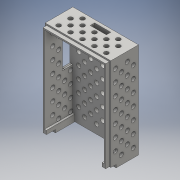
# Autodesk Inventor part: RaspPiCaseBottom
Saved by Autodesk Inventor 2016 (Build 200138000, 138)
## iProperties
Created: 2016-04-29
Part Number: RaspPiCaseBottom
Material: Generic
Document SubType Name: Modeling
Designer: mkepler
Density: 1 g/cm^3
Appearance: Default
Author: mkepler
Autodesk Inventor part; units mm, degrees
ref_plane "YZ Plane" through (0, 0, 0) normal (1, 0, 0) x (0, 1, 0)
ref_plane "XZ Plane" through (0, 0, 0) normal (0, 1, 0) x (-1, 0, 0)
ref_plane "XY Plane" through (0, 0, 0) normal (0, 0, 1) x (1, 0, 0)
sketch "Sketch1" plane through (0, 0, 0) normal (0, 1, 0) x (-1, 0, 0)
  line L0 (0, 0) -> (60, 0)
  line L1 (60, 0) -> (60, -90)
  line L2 (60, -90) -> (0, -90)
  line L3 (0, -90) -> (0, 0)
  circle A0 centre (6, -6) radius 2.15
  circle A1 centre (12, -12) radius 2.15
  line L4 (0, 0) -> (15, 0)
  line L5 (15, -28.7108) -> (16.2859, -28.7108)
  circle A2 centre (24, -12) radius 2.15
  circle A3 centre (18, -6) radius 2.15
  line L6 (0, 0) -> (27, 0)
  circle A4 centre (48, -12) radius 2.15
  circle A5 centre (42, -6) radius 2.15
  circle A6 centre (30, -6) radius 2.15
  circle A7 centre (36, -12) radius 2.15
  circle A8 centre (54, -6) radius 2.15
  line L7 (60, 0) -> (60, -15)
  line L8 (60, 0) -> (60, -15)
  line L9 (60, -15) -> (56.15, -15)
  circle A9 centre (6, -18) radius 2.15
  circle A10 centre (12, -24) radius 2.15
  circle A11 centre (24, -24) radius 2.15
  circle A12 centre (18, -18) radius 2.15
  circle A13 centre (30, -18) radius 2.15
  circle A14 centre (36, -24) radius 2.15
  circle A15 centre (42, -18) radius 2.15
  circle A16 centre (48, -24) radius 2.15
  circle A17 centre (54, -18) radius 2.15
  line L10 (60, 0) -> (60, -27)
  circle A18 centre (6, -42) radius 2.15
  circle A19 centre (18, -42) radius 2.15
  circle A20 centre (30, -42) radius 2.15
  circle A21 centre (42, -42) radius 2.15
  circle A22 centre (54, -42) radius 2.15
  circle A23 centre (54, -30) radius 2.15
  circle A24 centre (48, -36) radius 2.15
  circle A25 centre (42, -30) radius 2.15
  circle A26 centre (36, -36) radius 2.15
  circle A27 centre (30, -30) radius 2.15
  circle A28 centre (24, -36) radius 2.15
  circle A29 centre (18, -30) radius 2.15
  circle A30 centre (12, -36) radius 2.15
  circle A31 centre (6, -30) radius 2.15
  line L11 (60, 0) -> (60, -45)
  line L12 (60, -45) -> (48.8128, -45)
  circle A32 centre (6, -78) radius 2.15
  circle A33 centre (12, -84) radius 2.15
  line L13 (15, -61.2892) -> (16.2859, -61.2892)
  circle A34 centre (24, -84) radius 2.15
  circle A35 centre (18, -78) radius 2.15
  circle A36 centre (30, -78) radius 2.15
  circle A37 centre (36, -84) radius 2.15
  circle A38 centre (42, -78) radius 2.15
  circle A39 centre (48, -84) radius 2.15
  circle A40 centre (54, -78) radius 2.15
  line L14 (60, -75) -> (56.15, -75)
  circle A41 centre (54, -66) radius 2.15
  circle A42 centre (48, -72) radius 2.15
  circle A43 centre (42, -66) radius 2.15
  circle A44 centre (36, -72) radius 2.15
  circle A45 centre (30, -66) radius 2.15
  circle A46 centre (24, -72) radius 2.15
  circle A47 centre (18, -66) radius 2.15
  circle A48 centre (12, -72) radius 2.15
  circle A49 centre (6, -66) radius 2.15
  circle A50 centre (54, -54) radius 2.15
  circle A51 centre (48, -60) radius 2.15
  circle A52 centre (48, -48) radius 2.15
  circle A53 centre (42, -54) radius 2.15
  circle A54 centre (36, -60) radius 2.15
  circle A55 centre (36, -48) radius 2.15
  circle A56 centre (30, -54) radius 2.15
  circle A57 centre (24, -60) radius 2.15
  circle A58 centre (24, -48) radius 2.15
  circle A59 centre (18, -54) radius 2.15
  circle A60 centre (12, -60) radius 2.15
  circle A61 centre (12, -48) radius 2.15
  circle A62 centre (6, -54) radius 2.15
  dimension "d0" = 60
  dimension "d1" = 4.3
  dimension "d2" = 6
  dimension "d3" = 6
  dimension "d6" = 90
  dimension "d7" = 4.3
  dimension "d10" = 15
  dimension "d12" = 27
  dimension "d13" = 4.3
  dimension "d17" = 15
  dimension "d18" = 27
  dimension "d19" = 45
  constraints: 63 centre point, 30 end point, 4 point on line, 4 symmetric about line, 2 horizontal, 2 parallel, 2 perpendicular, 1 collinear, 1 midpoint
  measures "d0" distance of L1.end L2.end
  measures "d1" diameter of A0
  measures "d2" distance from line of L0 A0.centre
  measures "d3" distance from line of L3 A0.centre
  measures "d6" distance of L0.end L1.end
  measures "d7" diameter of A1
  measures "d10" distance of L0.start L4.end
  measures "d12" distance of L0.start L6.end
  measures "d13" diameter of A8
  measures "d17" distance of L0.end L7.end
  measures "d18" distance of L0.end L10.end
  measures "d19" distance of L0.end L11.end
extrude "Extrusion1" add sketch "Sketch1" along normal blind 1.5
sketch "Sketch3" plane through (0, 0, 0) normal (1, 0, 0) x (0, 0, -1)
  line L0 (0, 1.5) -> (90, 1.5) projected
  line L1 (0, 1.5) -> (90, 1.5)
  line L2 (90, 1.5) -> (90, -28.5)
  line L3 (90, -28.5) -> (0, -28.5)
  line L4 (0, -28.5) -> (0, 1.5)
  point P0 (0, 0)
  dimension "d25" = 90
  dimension "d26" = 30
  constraints: 8 end point, 2 parallel, 1 horizontal, 1 perpendicular
  measures "d25" distance of L2.end L3.end
  measures "d26" distance of L1.end L2.end
extrude "Extrusion3" add sketch "Sketch3" along normal blind 1.5
sketch "Sketch5" plane through (-60, 0, -90) normal (-1, 0, 0) x (0, 0, 1)
  line L0 (90, -28.5) -> (90, 0) projected
  line L1 (90, 1.5) -> (0, 1.5)
  line L2 (0, 1.5) -> (0, -28.5)
  line L3 (0, -28.5) -> (90, -28.5)
  line L4 (90, -28.5) -> (90, 1.5)
  dimension "d31" = 90
  dimension "d32" = 30
  constraints: 8 end point, 2 parallel, 1 horizontal, 1 perpendicular
  measures "d31" distance of L3.end L2.end
  measures "d32" distance of L2.end L1.end
extrude "Extrusion5" add sketch "Sketch5" along normal blind 1.5
sketch "Sketch8" plane through (0, 1.5, 0) normal (0, 1, 0) x (1, 0, 0)
  line L0 (-61.5, 0) -> (-61.5, 90) projected
  line L1 (-61.5, 0) -> (1.5, 0)
  line L2 (1.5, 0) -> (1.5, -1.5)
  line L3 (1.5, -1.5) -> (-61.5, -1.5)
  line L4 (-61.5, -1.5) -> (-61.5, 0)
  point P0 (0, 0)
  dimension "d40" = 63
  dimension "d41" = 1.5
  constraints: 8 end point, 2 parallel, 1 horizontal, 1 perpendicular
  measures "d40" distance of L2.end L3.end
  measures "d41" distance of L1.end L2.end
extrude "Extrusion7" add sketch "Sketch8" against normal blind 30
sketch "Sketch9" plane through (-61.5, 0, -90) normal (-1, 0, 0) x (0, 0, 1)
  line L0 (91.5, 1.5) -> (91.5, -28.5) projected
  circle A0 centre (84, -8.3) radius 2.15
  line L1 (84, -2.3) -> (84, -8.3)
  line L2 (91.5, 1.5) -> (91.5, -28.5) projected
  line L3 (84, -8.3) -> (84, -11.3)
  line L4 (84, -11.3) -> (91.5, -11.3)
  circle A1 centre (84, -20.3) radius 2.15
  line L5 (84, -20.3) -> (84, -14.3)
  line L6 (84, -14.3) -> (84, -11.3)
  line L7 (81, -2.3) -> (81, -28.5)
  circle A2 centre (78, -2.3) radius 2.15
  line L8 (78, -2.3) -> (78, -8.3)
  line L9 (78, -8.3) -> (78, -11.3)
  line L10 (78, -11.3) -> (70.5, -11.3)
  circle A3 centre (78, -14.3) radius 2.15
  line L11 (78, -20.3) -> (78, -14.3)
  line L12 (78, -14.3) -> (78, -11.3)
  line L13 (78, -2.3) -> (81, -2.3)
  line L14 (78, -20.3) -> (75, -20.3)
  line L15 (75, -20.3) -> (75, -8.9833)
  circle A4 centre (66, -2.3) radius 2.15
  line L16 (66, -11.3) -> (58.5, -11.3)
  circle A5 centre (66, -14.3) radius 2.15
  line L17 (69, -2.3) -> (69, -28.5)
  line L18 (72, -11.3) -> (79.5, -11.3)
  circle A6 centre (72, -8.3) radius 2.15
  circle A7 centre (72, -20.3) radius 2.15
  line L19 (72, -20.3) -> (75, -20.3)
  line L20 (66, -20.3) -> (63, -20.3)
  line L21 (63, -20.3) -> (63, -15.4)
  circle A8 centre (42, -2.3) radius 2.15
  line L22 (42, -2.3) -> (42, -8.3)
  line L23 (42, -8.3) -> (42, -11.3)
  circle A9 centre (42, -14.3) radius 2.15
  line L24 (42, -20.3) -> (42, -14.3)
  line L25 (42, -14.3) -> (42, -11.3)
  line L26 (42, -2.3) -> (45, -2.3)
  line L27 (48, -2.3) -> (48, -8.3)
  line L28 (48, -2.3) -> (45, -2.3)
  line L29 (48, -11.3) -> (55.5, -11.3)
  line L30 (48, -8.3) -> (48, -11.3)
  circle A10 centre (48, -8.3) radius 2.15
  line L31 (48, -14.3) -> (48, -11.3)
  line L32 (48, -20.3) -> (48, -14.3)
  circle A11 centre (48, -20.3) radius 2.15
  line L33 (48, -20.3) -> (51, -20.3)
  line L34 (51, -20.3) -> (51, -8.9833)
  circle A12 centre (54, -14.3) radius 2.15
  line L35 (54, -20.3) -> (51, -20.3)
  circle A13 centre (60, -20.3) radius 2.15
  circle A14 centre (60, -8.3) radius 2.15
  line L36 (54, -11.3) -> (46.5, -11.3)
  circle A15 centre (54, -2.3) radius 2.15
  line L37 (42, -20.3) -> (39, -20.3)
  line L38 (39, -20.3) -> (39, -14.6416)
  circle A16 centre (6, -14.3) radius 2.15
  circle A17 centre (12, -20.3) radius 2.15
  circle A18 centre (12, -8.3) radius 2.15
  circle A19 centre (6, -2.3) radius 2.15
  line L39 (12, -20.3) -> (15, -20.3)
  line L40 (15, -20.3) -> (15, -15.4)
  circle A20 centre (24, -20.3) radius 2.15
  line L41 (30, -20.3) -> (27, -20.3)
  line L42 (30, -20.3) -> (30, -14.3)
  line L43 (30, -11.3) -> (22.5, -11.3)
  line L44 (30, -14.3) -> (30, -11.3)
  line L45 (24, -11.3) -> (31.5, -11.3)
  circle A21 centre (30, -14.3) radius 2.15
  line L46 (30, -8.3) -> (30, -11.3)
  line L47 (36, -20.3) -> (36, -14.3)
  circle A22 centre (36, -20.3) radius 2.15
  line L48 (24, -20.3) -> (27, -20.3)
  line L49 (30, -2.3) -> (30, -8.3)
  line L50 (30, -2.3) -> (33, -2.3)
  circle A23 centre (30, -2.3) radius 2.15
  circle A24 centre (36, -8.3) radius 2.15
  line L51 (36, -2.3) -> (36, -8.3)
  line L52 (36, -8.3) -> (36, -11.3)
  line L53 (36, -14.3) -> (36, -11.3)
  line L54 (36, -2.3) -> (33, -2.3)
  circle A25 centre (24, -8.3) radius 2.15
  circle A26 centre (18, -2.3) radius 2.15
  circle A27 centre (18, -14.3) radius 2.15
  line L55 (36, -20.3) -> (39, -20.3)
  point P0 (90, 0)
  point P1 (66, -8.3)
  point P2 (72, -2.3)
  point P3 (60, -2.3)
  point P4 (60, -14.3)
  point P5 (57, -2.3)
  point P6 (60, -11.3)
  point P7 (54, -8.3)
  point P8 (12, -2.3)
  point P9 (12, -14.3)
  point P10 (6, -20.3)
  point P11 (6, -8.3)
  point P12 (18, -20.3)
  point P13 (24, -14.3)
  point P14 (18, -11.3)
  point P15 (18, -8.3)
  point P16 (24, -2.3)
  point P17 (21, -2.3)
  dimension "d46" = 7.5
  dimension "d47" = 4.3
  dimension "d48" = 6
  dimension "d49" = 3
  dimension "d50" = 3
  dimension "d51" = 3
  dimension "d52" = 3
  dimension "d53" = 3
  constraints: 108 end point, 80 symmetric about line, 28 centre point, 13 point on line, 3 horizontal, 3 perpendicular, 1 parallel, 1 vertical
  measures "d46" distance from line of L0 L1.start
  measures "d47" diameter of A0
  measures "d48" distance of L1.start L1.end
  measures "d49" distance of L1.end L3.end
  measures "d50" distance of L1.start L7.start
  measures "d51" distance of L11.start L14.end
  measures "d52" distance of L20.start L20.end
  measures "d53" distance of L24.start L37.end
sketch "Sketch10" plane through (-61.5, 1.5, 1.5) normal (0, 0, 1) x (1, 0, 0)
  line L0 (63, 0) -> (0, 0) projected
  line L1 (0, 0) -> (0, -30) projected
  circle A0 centre (13.5, -3.8) radius 2.15
  circle A1 centre (7.5, -9.8) radius 2.15
  line L2 (7.5, -9.8) -> (7.5, -12.8)
  line L3 (7.5, -12.8) -> (8.9551, -12.8)
  circle A2 centre (7.5, -21.8) radius 2.15
  circle A3 centre (13.5, -15.8) radius 2.15
  line L4 (7.5, -15.8) -> (7.5, -12.8)
  line L5 (13.5, -3.8) -> (16.5, -3.8)
  line L6 (16.5, -3.8) -> (16.5, -8.3155)
  circle A4 centre (25.5, -3.8) radius 2.15
  circle A5 centre (19.5, -9.8) radius 2.15
  line L7 (25.5, -9.8) -> (25.5, -12.8)
  line L8 (25.5, -12.8) -> (24.0449, -12.8)
  circle A6 centre (19.5, -21.8) radius 2.15
  circle A7 centre (25.5, -15.8) radius 2.15
  line L9 (25.5, -15.8) -> (25.5, -12.8)
  line L10 (19.5, -3.8) -> (16.5, -3.8)
  line L11 (25.5, -3.8) -> (28.5, -3.8)
  line L12 (28.5, -3.8) -> (28.5, -7.65)
  circle A8 centre (49.5, -3.8) radius 2.15
  circle A9 centre (43.5, -9.8) radius 2.15
  line L13 (49.5, -9.8) -> (49.5, -12.8)
  line L14 (49.5, -12.8) -> (48.0449, -12.8)
  circle A10 centre (43.5, -21.8) radius 2.15
  circle A11 centre (49.5, -15.8) radius 2.15
  line L15 (49.5, -15.8) -> (49.5, -12.8)
  line L16 (43.5, -3.8) -> (40.5, -3.8)
  line L17 (40.5, -3.8) -> (40.5, -8.3155)
  line L18 (31.5, -12.8) -> (32.9551, -12.8)
  line L19 (31.5, -15.8) -> (31.5, -12.8)
  circle A12 centre (37.5, -15.8) radius 2.15
  circle A13 centre (31.5, -21.8) radius 2.15
  line L20 (31.5, -9.8) -> (31.5, -12.8)
  circle A14 centre (31.5, -9.8) radius 2.15
  line L21 (37.5, -3.8) -> (40.5, -3.8)
  circle A15 centre (37.5, -3.8) radius 2.15
  line L22 (49.5, -3.8) -> (52.5, -3.8)
  line L23 (52.5, -3.8) -> (52.5, -9.251)
  circle A16 centre (55.5, -9.8) radius 2.15
  line L24 (55.5, -9.8) -> (55.5, -12.8)
  line L25 (55.5, -12.8) -> (56.9551, -12.8)
  circle A17 centre (55.5, -21.8) radius 2.15
  line L26 (55.5, -15.8) -> (55.5, -12.8)
  line L27 (55.5, -3.8) -> (52.5, -3.8)
  point P0 (61.5, -1.5)
  point P1 (7.5, -3.8)
  point P2 (13.5, -9.8)
  point P3 (13.5, -21.8)
  point P4 (25.5, -21.8)
  point P5 (19.5, -15.8)
  point P6 (43.5, -15.8)
  point P7 (37.5, -21.8)
  point P8 (37.5, -9.8)
  point P9 (31.5, -3.8)
  dimension "d62" = 3.8
  dimension "d63" = 7.5
  dimension "d64" = 4.3
  dimension "d65" = 6
  dimension "d66" = 4.3
  dimension "d67" = 6
  dimension "d69" = 3
  dimension "d70" = 3
  dimension "d71" = 3
  dimension "d72" = 3
  constraints: 52 end point, 40 symmetric about line, 18 centre point, 4 horizontal, 3 perpendicular, 1 vertical
  measures "d62" distance from line of L0 point (7.5, -3.8)
  measures "d63" distance from line of L1 point (7.5, -3.8)
  measures "d64" diameter of A0
  measures "d65" distance of L5.start point (7.5, -3.8)
  measures "d66" diameter of A1
  measures "d67" distance of L2.start point (7.5, -3.8)
  measures "d69" distance of L2.start L2.end
  measures "d70" distance of L5.start L5.end
  measures "d71" distance of L11.start L11.end
  measures "d72" distance of L22.start L22.end
sketch "Sketch11" plane through (-61.5, 1.5, 1.5) normal (0, 0, 1) x (1, 0, 0)
  line L0 (1.5, -1.5) -> (61.5, -1.5) projected
  line L1 (39.65, -1.5) -> (23.1579, -1.5)
  line L2 (23.1579, -1.5) -> (23.1579, -5.95)
  line L3 (23.1579, -5.95) -> (39.65, -5.95)
  line L4 (39.65, -5.95) -> (39.65, -1.5)
  constraints: 8 end point, 2 parallel, 1 horizontal, 1 perpendicular, 1 point on line
extrude "Extrusion8" cut sketch "Sketch11" against normal blind 30
sketch "Sketch12" plane through (-60, 0, -90) normal (1, 0, 0) x (0, 0, -1)
  line L0 (0, 0) -> (-90, 0) projected
  line L1 (0, -28.5) -> (-90, -28.5) projected
  line L2 (0, 0) -> (-3.7, 0)
  line L3 (-3.7, 0) -> (-3.7, -28.5)
  line L4 (-3.7, -28.5) -> (0, -28.5)
  line L5 (0, -28.5) -> (0, 0)
  dimension "d82" = 3.7
  constraints: 8 end point, 2 parallel, 1 horizontal, 1 perpendicular, 1 point on line
  measures "d82" distance of L4.end L3.end
extrude "Extrusion9" add sketch "Sketch12" along normal blind 2
sketch "Sketch13" plane through (0, 0, 0) normal (-1, 0, 0) x (0, 0, 1)
  line L0 (-90, -28.5) -> (0, -28.5) projected
  line L1 (-90, 0) -> (-86.3, 0)
  line L2 (-86.3, 0) -> (-86.3, -28.5)
  line L3 (-86.3, -28.5) -> (-90, -28.5)
  line L4 (-90, -28.5) -> (-90, 0)
  point P0 (0, 0)
  dimension "d85" = 3.7
  constraints: 8 end point, 2 parallel, 1 horizontal, 1 perpendicular, 1 point on line
  measures "d85" distance of L2.end L3.end
extrude "Extrusion10" add sketch "Sketch13" along normal blind 2
sketch "Sketch14" plane through (0, 0, 0) normal (-1, 0, 0) x (0, 0, 1)
  point P0 (0, 0)
sketch "Sketch16" plane through (0, 0, 0) normal (0, -1, 0) x (1, 0, 0)
  point P0 (0, 0)
hole "Hole3" at (-61.5, -20.3, -6) at (-61.5, -14.3, -12) at (-61.5, -20.3, -18) at (-61.5, -14.3, -24) at (-61.5, -8.3, -6) at (-61.5, -2.3, -12) at (-61.5, -8.3, -18) at (-61.5, -2.3, -24) at (-61.5, -8.3, -30) at (-61.5, -20.3, -30) at (-61.5, -14.3, -36) at (-61.5, -2.3, -36) at (-61.5, -8.3, -42) at (-61.5, -20.3, -42) at (-61.5, -14.3, -48) at (-61.5, -20.3, -54) at (-61.5, -8.3, -54) at (-61.5, -2.3, -48) at (-61.5, -2.3, -60) at (-61.5, -14.3, -60) at (-61.5, -8.3, -66) at (-61.5, -8.3, -78) at (-61.5, -14.3, -72) at (-61.5, -20.3, -66) at (-61.5, -2.3, -72) at (-61.5, -2.3, -84) at (-61.5, -14.3, -84) at (-61.5, -20.3, -78) direction (1, 0, 0) diameter 4.35 end through all
hole "Hole4" at (-6, -20.3, 1.5) at (-18, -20.3, 1.5) at (-30, -20.3, 1.5) at (-42, -20.3, 1.5) at (-54, -20.3, 1.5) at (-48, -14.3, 1.5) at (-36, -14.3, 1.5) at (-24, -14.3, 1.5) at (-12, -14.3, 1.5) at (-6, -8.3, 1.5) at (-18, -8.3, 1.5) at (-12, -2.3, 1.5) at (-30, -8.3, 1.5) at (-42, -8.3, 1.5) at (-48, -2.3, 1.5) at (-54, -8.3, 1.5) direction (0, 0, -1) diameter 4.35 end through all
sketch "Sketch17" plane through (-61.5, 0, -90) normal (-1, 0, 0) x (0, 0, 1)
  line L0 (86.15, 0) -> (81.85, 0) projected
  line L1 (86.15, 0) -> (86.15, -10.475)
  line L2 (86.15, -10.475) -> (45.825, -10.475)
  line L3 (45.825, -10.475) -> (45.85, 0)
  line L4 (45.85, 0) -> (45.85, 1.5) projected
  line L5 (50.15, 0) -> (45.85, 0) projected
  line L6 (86.15, 0) -> (45.85, 0)
  point P0 (90, 0)
  constraints: 8 end point, 1 horizontal, 1 perpendicular, 1 point on line, 1 vertical
extrude "Extrusion12" cut sketch "Sketch17" against normal blind 10
sketch "Sketch18" plane through (-61.5, 0, -90) normal (-1, 0, 0) x (0, 0, 1)
  line L0 (91.5, 1.5) -> (91.5, -28.5) projected
  line L1 (91.5, -28.5) -> (91.5, -24.85)
  line L2 (91.5, -24.85) -> (0, -24.85)
  line L3 (0, -28.5) -> (0, 0) projected
  line L4 (91.5, 1.5) -> (0, 1.5) projected
  line L5 (0, 1.5) -> (91.5, 1.5)
  line L6 (91.5, 1.5) -> (91.5, -24.85)
  line L7 (0, 1.5) -> (0, -24.85)
  circle A0 centre (84, -20.3) radius 2.175 projected
  circle A1 centre (84, -20.3) radius 2.175
  circle A2 centre (66, -14.3) radius 2.175 projected
  circle A3 centre (66, -14.3) radius 2.175
  circle A4 centre (72, -20.3) radius 2.175 projected
  circle A5 centre (72, -20.3) radius 2.175
  circle A6 centre (60, -20.3) radius 2.175 projected
  circle A7 centre (60, -20.3) radius 2.175
  circle A8 centre (54, -14.3) radius 2.175 projected
  circle A9 centre (54, -14.3) radius 2.175
  circle A10 centre (48, -20.3) radius 2.175 projected
  circle A11 centre (48, -20.3) radius 2.175
  circle A12 centre (36, -20.3) radius 2.175 projected
  circle A13 centre (36, -20.3) radius 2.175
  circle A14 centre (42, -14.3) radius 2.175 projected
  circle A15 centre (42, -14.3) radius 2.175
  circle A16 centre (78, -14.3) radius 2.175 projected
  circle A17 centre (78, -14.3) radius 2.175
  circle A18 centre (42, -2.3) radius 2.175 projected
  circle A19 centre (42, -2.3) radius 2.175
  circle A20 centre (36, -8.3) radius 2.175 projected
  circle A21 centre (36, -8.3) radius 2.175
  circle A22 centre (30, -2.3) radius 2.175 projected
  circle A23 centre (30, -2.3) radius 2.175
  circle A24 centre (24, -8.3) radius 2.175 projected
  circle A25 centre (24, -8.3) radius 2.175
  circle A26 centre (24, -20.3) radius 2.175 projected
  circle A27 centre (24, -20.3) radius 2.175
  circle A28 centre (6, -14.3) radius 2.175 projected
  circle A29 centre (6, -14.3) radius 2.175
  circle A30 centre (12, -8.3) radius 2.175 projected
  circle A31 centre (12, -8.3) radius 2.175
  circle A32 centre (6, -2.3) radius 2.175
  circle A33 centre (18, -2.3) radius 2.175
  line L8 (90, 0) -> (3.7, 0) projected
  line L9 (86.175, 0) -> (45.825, 0)
  line L10 (45.825, 0) -> (45.825, -10.475)
  line L11 (45.825, -10.475) -> (86.175, -10.475)
  line L12 (86.175, -10.475) -> (86.175, 0)
  circle A34 centre (30, -14.3) radius 2.175
  circle A35 centre (18, -14.3) radius 2.175
  circle A36 centre (12, -20.3) radius 2.175
  dimension "d116" = 3.65
  dimension "d117" = 4.35
  dimension "d118" = 4.35
  dimension "d119" = 4.35
  dimension "d120" = 4.35
  dimension "d121" = 4.35
  dimension "d122" = 4.35
  dimension "d123" = 4.35
  dimension "d124" = 4.35
  dimension "d125" = 4.35
  dimension "d126" = 4.35
  constraints: 21 centre point, 18 end point, 16 coincident, 3 perpendicular, 3 point on line, 2 collinear, 2 parallel, 1 horizontal
  measures "d116" distance of L0.end L1.end
  measures "d117" diameter of A1
  measures "d118" diameter of A3
  measures "d119" diameter of A5
  measures "d120" diameter of A7
  measures "d121" diameter of A9
  measures "d122" diameter of A11
  measures "d123" diameter of A13
  measures "d124" diameter of A15
  measures "d125" diameter of A23
  measures "d126" diameter of A25
extrude "Extrusion13" add sketch "Sketch18" along normal blind 1.5
sketch "Sketch19" plane through (-61.5, -28.5, 1.5) normal (0, 0, 1) x (1, 0, 0)
  point P0 (61.5, 28.5)
sketch "Sketch20" plane through (1.5, 0, 0) normal (1, 0, 0) x (0, 0, -1)
  line L0 (-1.5, -24.85) -> (90, -24.85) projected
  line L1 (-1.5, -24.85) -> (-1.5, -28.5) projected
  line L2 (90, -24.85) -> (-1.5, -24.85)
  line L3 (-1.5, -24.85) -> (-1.5, 1.5) projected
  line L4 (-1.5, -24.85) -> (-1.5, 1.5)
  line L5 (-1.5, 1.5) -> (90, 1.5) projected
  line L6 (-1.5, 1.5) -> (90, 1.5)
  line L7 (90, 1.5) -> (90, -24.85)
  line L8 (90, -28.5) -> (90, 0) projected
  circle A0 centre (78.0652, -20.3438) radius 2.175
  circle A1 centre (84, -14.3) radius 2.175 projected
  circle A2 centre (84, -14.3) radius 2.175
  circle A3 centre (72, -2.3) radius 2.175 projected
  circle A4 centre (72, -2.3) radius 2.175
  circle A5 centre (84, -2.3) radius 2.175
  circle A6 centre (72, -14.3) radius 2.175
  circle A7 centre (66, -20.3) radius 2.175 projected
  circle A8 centre (66, -20.3) radius 2.175
  circle A9 centre (66, -8.3) radius 2.175
  circle A10 centre (60, -2.3) radius 2.175 projected
  circle A11 centre (60, -2.3) radius 2.175
  circle A12 centre (60, -14.3) radius 2.175 projected
  circle A13 centre (60, -14.3) radius 2.175
  circle A14 centre (54, -20.3) radius 2.175 projected
  circle A15 centre (54, -20.3) radius 2.175
  circle A16 centre (54, -8.3) radius 2.175
  circle A17 centre (48, -2.3) radius 2.175 projected
  circle A18 centre (48, -2.3) radius 2.175
  circle A19 centre (48, -14.3) radius 2.175
  circle A20 centre (42, -20.3) radius 2.175 projected
  circle A21 centre (42, -20.3) radius 2.175
  circle A22 centre (42, -8.3) radius 2.175 projected
  circle A23 centre (42, -8.3) radius 2.175
  circle A24 centre (36, -2.3) radius 2.175 projected
  circle A25 centre (36, -2.3) radius 2.175
  circle A26 centre (30, -20.3) radius 2.175 projected
  circle A27 centre (30, -20.3) radius 2.175
  circle A28 centre (36, -14.3) radius 2.175 projected
  circle A29 centre (36, -14.3) radius 2.175
  circle A30 centre (30, -8.3) radius 2.175
  circle A31 centre (24, -14.3) radius 2.175 projected
  circle A32 centre (24, -14.3) radius 2.175
  circle A33 centre (24, -2.3) radius 2.175
  circle A34 centre (6, -8.3) radius 2.175 projected
  circle A35 centre (6, -8.3) radius 2.175
  circle A36 centre (12, -2.3) radius 2.175 projected
  circle A37 centre (12, -2.3) radius 2.175
  circle A38 centre (18, -8.3) radius 2.175 projected
  circle A39 centre (18, -8.3) radius 2.175
  circle A40 centre (12, -14.3) radius 2.175
  circle A41 centre (6, -20.3) radius 2.175
  circle A42 centre (18, -20.3) radius 2.175
  point P0 (0, 0)
  dimension "d129" = 4.35
  dimension "d130" = 4.35
  constraints: 27 centre point, 16 coincident, 8 end point, 3 collinear, 1 perpendicular
  measures "d129" diameter of A0
  measures "d130" diameter of A2
extrude "Extrusion14" add sketch "Sketch20" along normal blind 1.5
sketch "Sketch21" plane through (-61.5, -28.5, 1.5) normal (0, 0, 1) x (1, 0, 0)
  line L0 (63, 3.65) -> (64.5, 3.65) projected
  line L1 (0, 3.65) -> (-1.5, 3.65) projected
  line L2 (64.5, 3.65) -> (-1.5, 3.65)
  line L3 (-1.5, 3.65) -> (-1.5, 30) projected
  line L4 (-1.5, 3.65) -> (-1.5, 30)
  line L5 (-1.5, 30) -> (64.5, 30) projected
  line L6 (-1.5, 30) -> (64.5, 30)
  line L7 (64.5, 30) -> (64.5, 3.65) projected
  line L8 (64.5, 30) -> (64.5, 3.65)
  circle A0 centre (55.5, 8.2) radius 2.175 projected
  circle A1 centre (55.5, 8.2) radius 2.175
  circle A2 centre (49.5, 14.2) radius 2.175 projected
  circle A3 centre (49.5, 14.2) radius 2.175
  circle A4 centre (55.5, 20.2) radius 2.175 projected
  circle A5 centre (55.5, 20.2) radius 2.175
  circle A6 centre (49.5, 26.2) radius 2.175 projected
  circle A7 centre (49.5, 26.2) radius 2.175
  circle A8 centre (43.5, 20.2) radius 2.175 projected
  circle A9 centre (43.5, 20.2) radius 2.175
  circle A10 centre (43.5, 8.2) radius 2.175 projected
  circle A11 centre (43.5, 8.2) radius 2.175
  circle A12 centre (37.5, 14.2) radius 2.175 projected
  circle A13 centre (37.5, 14.2) radius 2.175
  circle A14 centre (31.5, 8.2) radius 2.175
  circle A15 centre (31.5, 20.2) radius 2.175
  circle A16 centre (19.5, 20.2) radius 2.175 projected
  circle A17 centre (19.5, 20.2) radius 2.175
  circle A18 centre (25.5, 14.2) radius 2.175 projected
  circle A19 centre (25.5, 14.2) radius 2.175
  circle A20 centre (7.5, 8.2) radius 2.175 projected
  circle A21 centre (7.5, 8.2) radius 2.175
  circle A22 centre (13.5, 14.2) radius 2.175 projected
  circle A23 centre (13.5, 14.2) radius 2.175
  circle A24 centre (7.5, 20.2) radius 2.175
  circle A25 centre (13.5, 26.2) radius 2.175
  line L9 (23.1579, 24.05) -> (39.65, 24.05) projected
  line L10 (27.65, 28.5) -> (23.35, 28.5) projected
  line L11 (39.65, 24.05) -> (23.35, 24.05)
  line L12 (23.35, 24.05) -> (23.35, 28.5)
  line L13 (23.35, 28.5) -> (39.65, 28.5)
  line L14 (39.65, 28.5) -> (39.65, 24.05)
  circle A26 centre (19.5, 8.2) radius 2.175
  point P0 (61.5, 28.5)
  constraints: 16 centre point, 16 end point, 11 coincident, 3 equal length, 3 perpendicular, 2 horizontal
sketch "Sketch22" plane through (0, 1.5, 0) normal (0, 1, 0) x (1, 0, 0)
  line L0 (1.5, 90) -> (3, 90) projected
  line L1 (-63, -3) -> (3, -3)
  line L2 (3, -3) -> (3, 90)
  line L3 (3, 90) -> (-63, 90)
  line L4 (-63, 90) -> (-63, -3)
  circle A0 centre (-54, 6) radius 2.15 projected
  circle A1 centre (-54, 6) radius 2.15
  circle A2 centre (-54, 18) radius 2.15 projected
  circle A3 centre (-54, 18) radius 2.15
  circle A4 centre (-54, 30) radius 2.15 projected
  circle A5 centre (-54, 30) radius 2.15
  circle A6 centre (-54, 54) radius 2.15 projected
  circle A7 centre (-54, 54) radius 2.15
  circle A8 centre (-54, 66) radius 2.15 projected
  circle A9 centre (-54, 66) radius 2.15
  circle A10 centre (-54, 78) radius 2.15 projected
  circle A11 centre (-54, 78) radius 2.15
  circle A12 centre (-48, 84) radius 2.15 projected
  circle A13 centre (-48, 84) radius 2.15
  circle A14 centre (-48, 72) radius 2.15 projected
  circle A15 centre (-48, 72) radius 2.15
  circle A16 centre (-48, 60) radius 2.15 projected
  circle A17 centre (-48, 60) radius 2.15
  circle A18 centre (-48, 48) radius 2.15 projected
  circle A19 centre (-48, 48) radius 2.15
  circle A20 centre (-48, 36) radius 2.15 projected
  circle A21 centre (-48, 36) radius 2.15
  circle A22 centre (-48, 24) radius 2.15 projected
  circle A23 centre (-48, 24) radius 2.15
  circle A24 centre (-48, 12) radius 2.15 projected
  circle A25 centre (-48, 12) radius 2.15
  circle A26 centre (-42, 6) radius 2.15 projected
  circle A27 centre (-42, 6) radius 2.15
  circle A28 centre (-42, 18) radius 2.15 projected
  circle A29 centre (-42, 18) radius 2.15
  circle A30 centre (-42, 30) radius 2.15 projected
  circle A31 centre (-42, 30) radius 2.15
  circle A32 centre (-54, 42) radius 2.15 projected
  circle A33 centre (-54, 42) radius 2.15
  circle A34 centre (-42, 42) radius 2.15 projected
  circle A35 centre (-42, 42) radius 2.15
  circle A36 centre (-42, 54) radius 2.15
  circle A37 centre (-42, 66) radius 2.15 projected
  circle A38 centre (-42, 66) radius 2.15
  circle A39 centre (-42, 78) radius 2.15 projected
  circle A40 centre (-42, 78) radius 2.15
  circle A41 centre (-36, 12) radius 2.15 projected
  circle A42 centre (-36, 12) radius 2.15
  circle A43 centre (-24, 12) radius 2.15 projected
  circle A44 centre (-24, 12) radius 2.15
  circle A45 centre (-30, 6) radius 2.15
  circle A46 centre (-30, 18) radius 2.15 projected
  circle A47 centre (-30, 18) radius 2.15
  circle A48 centre (-36, 24) radius 2.15 projected
  circle A49 centre (-36, 24) radius 2.15
  circle A50 centre (-36, 36) radius 2.15 projected
  circle A51 centre (-36, 36) radius 2.15
  circle A52 centre (-36, 48) radius 2.15 projected
  circle A53 centre (-36, 48) radius 2.15
  circle A54 centre (-36, 60) radius 2.15 projected
  circle A55 centre (-36, 60) radius 2.15
  circle A56 centre (-36, 72) radius 2.15
  circle A57 centre (-36, 84) radius 2.15
  circle A58 centre (-30, 78) radius 2.15 projected
  circle A59 centre (-30, 78) radius 2.15
  circle A60 centre (-30, 66) radius 2.15 projected
  circle A61 centre (-30, 66) radius 2.15
  circle A62 centre (-30, 54) radius 2.15 projected
  circle A63 centre (-30, 54) radius 2.15
  circle A64 centre (-30, 42) radius 2.15
  circle A65 centre (-30, 30) radius 2.15 projected
  circle A66 centre (-30, 30) radius 2.15
  circle A67 centre (-24, 24) radius 2.15 projected
  circle A68 centre (-24, 24) radius 2.15
  circle A69 centre (-24, 48) radius 2.15 projected
  circle A70 centre (-24, 48) radius 2.15
  circle A71 centre (-24, 60) radius 2.15 projected
  circle A72 centre (-24, 60) radius 2.15
  circle A73 centre (-24, 72) radius 2.15
  circle A74 centre (-24, 84) radius 2.15 projected
  circle A75 centre (-24, 84) radius 2.15
  circle A76 centre (-18, 78) radius 2.15 projected
  circle A77 centre (-18, 78) radius 2.15
  circle A78 centre (-18, 66) radius 2.15 projected
  circle A79 centre (-18, 66) radius 2.15
  circle A80 centre (-18, 54) radius 2.15
  circle A81 centre (-18, 42) radius 2.15 projected
  circle A82 centre (-18, 42) radius 2.15
  circle A83 centre (-24, 36) radius 2.15 projected
  circle A84 centre (-24, 36) radius 2.15
  circle A85 centre (-18, 30) radius 2.15 projected
  circle A86 centre (-18, 30) radius 2.15
  circle A87 centre (-18, 18) radius 2.15
  circle A88 centre (-18, 6) radius 2.15 projected
  circle A89 centre (-18, 6) radius 2.15
  circle A90 centre (-6, 6) radius 2.15 projected
  circle A91 centre (-6, 6) radius 2.15
  circle A92 centre (-12, 12) radius 2.15 projected
  circle A93 centre (-12, 12) radius 2.15
  circle A94 centre (-6, 18) radius 2.15 projected
  circle A95 centre (-6, 18) radius 2.15
  circle A96 centre (-12, 24) radius 2.15 projected
  circle A97 centre (-12, 24) radius 2.15
  circle A98 centre (-6, 30) radius 2.15 projected
  circle A99 centre (-6, 30) radius 2.15
  circle A100 centre (-12, 36) radius 2.15 projected
  circle A101 centre (-12, 36) radius 2.15
  circle A102 centre (-6, 42) radius 2.15 projected
  circle A103 centre (-6, 42) radius 2.15
  circle A104 centre (-12, 48) radius 2.15 projected
  circle A105 centre (-12, 48) radius 2.15
  circle A106 centre (-12, 60) radius 2.15 projected
  circle A107 centre (-12, 60) radius 2.15
  circle A108 centre (-6, 54) radius 2.15 projected
  circle A109 centre (-6, 54) radius 2.15
  circle A110 centre (-6, 78) radius 2.15 projected
  circle A111 centre (-6, 78) radius 2.15
  circle A112 centre (-12, 72) radius 2.15 projected
  circle A113 centre (-12, 72) radius 2.15
  circle A114 centre (-12, 84) radius 2.15 projected
  circle A115 centre (-12, 84) radius 2.15
  circle A116 centre (-6, 66) radius 2.15 projected
  circle A117 centre (-6, 66) radius 2.15
  point P0 (0, 0)
  constraints: 63 centre point, 55 coincident, 8 end point, 2 parallel, 1 horizontal, 1 perpendicular
extrude "Extrusion16" add sketch "Sketch22" along normal blind 1.5
sketch "Sketch23" plane through (-58, -28.5, -90) normal (0, 0, -1) x (-1, 0, 0)
  line L0 (0, 0) -> (0, 28.5) projected
  line L1 (0, 0) -> (0, 9)
  line L2 (0, 9) -> (5, 9)
  line L3 (5, 10.375) -> (5, 6.025) projected
  line L4 (5, 31.5) -> (-61, 31.5) projected
  line L5 (5, 9) -> (5, 31.5)
  line L6 (5, 31.5) -> (-61, 31.5)
  line L7 (-61, 31.5) -> (-61, 9)
  line L8 (-61, 6.025) -> (-61, 10.375) projected
  line L9 (-56, 0) -> (-56, 28.5) projected
  line L10 (-56, 9) -> (-56, 28.5)
  line L11 (-56, 28.5) -> (0, 28.5)
  line L12 (2, 28.5) -> (-19.6579, 28.5) projected
  line L13 (0, 9) -> (0, 28.5)
  line L14 (-61, 9) -> (-56, 9)
  point P0 (-58, 28.5)
  dimension "d137" = 9
  constraints: 18 end point, 4 collinear, 4 point on line, 1 horizontal, 1 perpendicular, 1 vertical
  measures "d137" distance of L0.start L1.end
extrude "Extrusion17" add sketch "Sketch23" along normal blind 3
extrude "Extrusion18" add sketch "Sketch21" along normal blind 1.5
sketch "Sketch24" plane through (3, 0, 0) normal (1, 0, 0) x (0, 0, -1)
  circle A0 centre (78, -8.3) radius 2.175 projected
  circle A1 centre (78, -8.3) radius 2.175
  point P0 (0, 0)
  constraints: 1 centre point, 1 coincident
hole "Hole5" at (3, -8.3, -78) direction (-1, 0, 0) diameter 4.35 end through all
body "Solid1"
